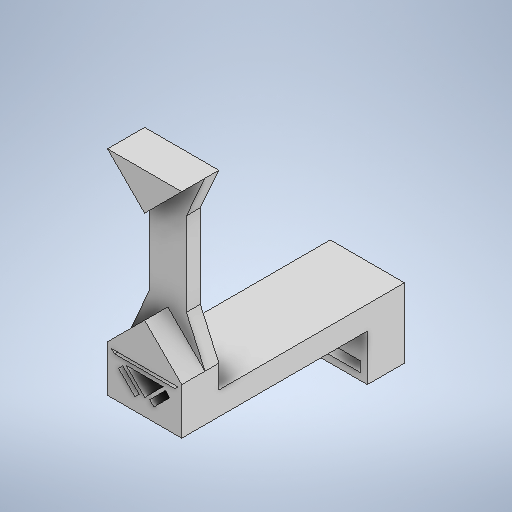
# Autodesk Inventor part: Connecting pt.2
Saved by Autodesk Inventor 2025.2 (Build 292293000, 293)
## iProperties
Created: 2025-04-14
Part Number: Connecting pt.2
Material: Generic
Document SubType Name: Modeling
Designer: 1khanhan2
Density: 1 g/cm^3
Appearance: Default
Author: 1khanhan2
Autodesk Inventor part; units mm, degrees
ref_plane "YZ Plane" through (0, 0, 0) normal (1, 0, 0) x (0, 1, 0)
ref_plane "XZ Plane" through (0, 0, 0) normal (0, 1, 0) x (-1, 0, 0)
ref_plane "XY Plane" through (0, 0, 0) normal (0, 0, 1) x (1, 0, 0)
sketch "Sketch1" plane through (0, 0, 0) normal (0, 0, 1) x (1, 0, 0)
  line L0 (0, 0) -> (0, 20)
  line L1 (0, 20) -> (16, 20)
  line L2 (16, 20) -> (16, 0)
  line L3 (16, 0) -> (0, 0)
  line L4 (8, 28) -> (0, 20)
  line L5 (8, 28) -> (16, 20)
  line L6 (0, 0) -> (0, 5)
  line L7 (0, 0) -> (0, 1.5)
  line L8 (0, 5) -> (0, 3.5)
  line L9 (1.5, 3.5) -> (1.5, 1.5)
  line L10 (1.5, 3.5) -> (14.5, 3.5)
  line L11 (14.5, 3.5) -> (14.5, 1.5)
  line L12 (14.5, 1.5) -> (1.5, 1.5)
  line L13 (14.5, 18.5) -> (15.1649, 19.1649)
  line L14 (15.1649, 19.1649) -> (0.8351, 19.1649)
  line L15 (0.8351, 19.1649) -> (1.5, 18.5)
  line L16 (1.5, 18.5) -> (14.5, 18.5)
  line L17 (12, 17.6183) -> (4, 17.6183)
  line L18 (4, 17.6183) -> (8.0319, 13.6184)
  line L19 (8.0319, 13.6184) -> (12, 17.6183)
  line L20 (12.4747, 17.1474) -> (13.3985, 16.231)
  line L21 (13.3985, 16.231) -> (10.016, 12.8213)
  line L22 (10.016, 12.8213) -> (9.0922, 13.7377)
  line L23 (9.0922, 13.7377) -> (12.4747, 17.1474)
  line L24 (6.8378, 13.6184) -> (3.2805, 17.1474)
  line L25 (3.2805, 17.1474) -> (2.3714, 16.231)
  line L26 (2.3714, 16.231) -> (5.9286, 12.702)
  line L27 (5.9286, 12.702) -> (6.8378, 13.6184)
  dimension "d0" = 20
  dimension "d1" = 16
  dimension "d3" = 5
  dimension "d7" = 1.5
  dimension "d9" = 13
  constraints: 56 end point, 14 perpendicular, 4 point on line, 2 horizontal, 1 parallel, 1 vertical
  measures "d0" distance of L0.start L0.end
  measures "d1" distance of L0.end L1.end
  measures "d3" distance of L0.start L6.end
  measures "d7" distance of L7.end L9.end
  measures "d9" distance of L9.start L10.end
extrude "Extrusion1" add sketch "Sketch1" along normal blind 5
extrude "Extrusion2" add sketch "Sketch1" along normal blind 4 contours L10 L11 L12 L9
sketch "Sketch2" plane through (0, 0, 0) normal (0, 0, -1) x (-1, 0, 0)
  line L0 (-16, 20) -> (-8, 28) projected
  line L1 (-16, 20) -> (0, 20)
  line L2 (0, 20) -> (-8, 28)
  line L3 (-16, 20) -> (-16, 56)
  line L4 (-16, 20) -> (20, 20) construction
  line L5 (-16, 56) -> (0, 56)
  line L6 (0, 56) -> (0, 20)
  line L7 (-16, 56) -> (-8, 48)
  line L8 (-16, 56) -> (-4.6863, 56) construction
  line L9 (-8, 48) -> (0, 56)
  point P0 (0, 0)
  dimension "d12" = 36
  dimension "d13" = 90
  dimension "d14" = 45
  constraints: 18 end point, 4 perpendicular, 3 horizontal, 2 equal length, 1 vertical
  measures "d12" distance of L0.start L3.end
  measures "d13" angle of L4 L3
  measures "d14" angle of L7 L8
extrude "Extrusion3" add sketch "Sketch2" against normal blind 5 contours L5 L9 L7
sketch "Sketch3" plane through (0, 0, 0) normal (0, 0, -1) x (-1, 0, 0)
  line L0 (0, 56) -> (-8, 48) projected
  line L1 (-16, 0) -> (-16, 20) projected
  line L2 (0, 56) -> (-16, 56)
  line L3 (-16, 56) -> (-16, 0)
  line L4 (-16, 0) -> (0, 0)
  line L5 (0, 0) -> (0, 56)
  line L6 (-16, 20) -> (-8, 28) projected
  line L7 (-16, 20) -> (0, 20)
  line L8 (-8, 28) -> (0, 20) projected
  line L9 (-8, 28) -> (-8, 48)
  line L10 (-16, 56) -> (-8, 38)
  line L11 (0, 56) -> (-8, 38)
  line L12 (-8, 38) -> (0, 20)
  line L13 (-8, 38) -> (-16, 20)
  line L14 (-12, 47) -> (-12, 29)
  line L15 (-4, 47) -> (-4, 29)
  point P0 (0, 0)
  constraints: 24 end point, 5 midpoint, 3 equal length, 3 perpendicular, 1 horizontal, 1 point on line
extrude "Extrusion4" add sketch "Sketch3" along normal blind 3 contours L11 L9 L0 | L0 L9 L10 L2 | L5 L4 L1 L7 | L7 L6 L8 | L8 L9 L12 | L15 L12 L11 | L13 L14 L10 | L9 L6 L13
sketch "Sketch4" plane through (0, 0, 5) normal (0, 0, 1) x (1, 0, 0)
  line L0 (0, 0) -> (0, 20) projected
  line L1 (16, 20) -> (16, 0) projected
  line L2 (0, 0) -> (16, 0)
  line L3 (16, 0) -> (16, 10)
  line L4 (16, 10) -> (0, 10)
  line L5 (0, 10) -> (0, 0)
  constraints: 8 end point, 2 parallel, 1 horizontal, 1 midpoint, 1 perpendicular
extrude "Extrusion5" cut sketch "Sketch4" against normal blind 10
sketch "Sketch5" plane through (0, 0, -3) normal (0, 0, -1) x (-1, 0, 0)
  line L0 (0, 10) -> (-16, 10) projected
  line L1 (0, 10) -> (0, 20) projected
  line L2 (-16, 10) -> (0, 10)
  line L3 (0, 10) -> (0, 15)
  line L4 (0, 15) -> (-16, 15)
  line L5 (-16, 15) -> (-16, 10)
  point P0 (0, 0)
  dimension "d21" = 5
  constraints: 8 end point, 2 parallel, 1 horizontal, 1 midpoint, 1 perpendicular
  measures "d21" distance of L3.end L2.end
extrude "Extrusion6" add sketch "Sketch5" along normal blind 40
sketch "Sketch6" plane through (0, 10, 5) normal (0, -1, 0) x (1, 0, 0)
  line L0 (16, -48) -> (0, -48) projected
  line L1 (16, 0) -> (16, -48) projected
  line L2 (0, -48) -> (16, -48)
  line L3 (16, -48) -> (16, -40)
  line L4 (16, -40) -> (0, -40)
  line L5 (0, -40) -> (0, -48)
  point P0 (0, -5)
  dimension "d24" = 8
  constraints: 8 end point, 2 parallel, 1 horizontal, 1 perpendicular, 1 point on line
  measures "d24" distance of L3.end L2.end
extrude "Extrusion7" add sketch "Sketch6" along normal blind 10
sketch "Sketch7" plane through (0, 10, -35) normal (0, 0, 1) x (1, 0, 0)
  line L0 (0, -10) -> (16, -10)
  line L1 (16, -10) -> (16, -5)
  line L2 (16, -5) -> (0, -5)
  line L3 (0, -5) -> (0, -10)
  line L4 (0, -10) -> (1.5, -10)
  line L5 (1.5, -10) -> (1.5, -8.5)
  line L6 (1.5, -8.5) -> (0, -8.5)
  line L7 (0, -8.5) -> (0, -10)
  line L8 (1.5, -8.5) -> (14.5, -8.5)
  line L9 (14.5, -8.5) -> (14.5, -6.3)
  line L10 (14.5, -6.3) -> (1.5, -6.3)
  line L11 (1.5, -6.3) -> (1.5, -8.5)
  dimension "d27" = 16
  dimension "d28" = 5
  dimension "d29" = 1.5
  dimension "d30" = 1.5
  dimension "d31" = 13
  dimension "d32" = 2.2
  constraints: 24 end point, 6 parallel, 3 horizontal, 3 perpendicular
  measures "d27" distance of L2.end L1.end
  measures "d28" distance of L1.end L0.end
  measures "d29" distance of L6.end L5.end
  measures "d30" distance of L5.end L4.end
  measures "d31" distance of L10.end L9.end
  measures "d32" distance of L9.end L8.end
extrude "Extrusion8" cut sketch "Sketch7" against normal blind 3 contours L11 L10 L9 L8
body "Solid1"
